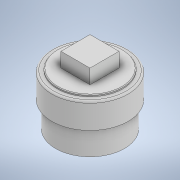
# Autodesk Inventor part: 4in Cleanout Adapter w Plug
Saved by Autodesk Inventor 2020 (Build 240168000, 168)
## iProperties
Created: 2020-01-08
Part Number: 4in Cleanout Adapter w Plug
Material: Generic
Document SubType Name: Modeling
Designer: ellio
Density: 1 g/cm^3
Appearance: Default
Author: ellio
Autodesk Inventor part; units mm, degrees
ref_plane "YZ Plane" through (0, 0, 0) normal (1, 0, 0) x (0, 1, 0)
ref_plane "XZ Plane" through (0, 0, 0) normal (0, 1, 0) x (-1, 0, 0)
ref_plane "XY Plane" through (0, 0, 0) normal (0, 0, 1) x (1, 0, 0)
sketch "Sketch1" plane through (0, 0, 0) normal (0, 1, 0) x (-1, 0, 0)
  circle A0 centre (0, 0) radius 53.975
  circle A1 centre (0, 0) radius 60.325
  dimension "d0" = 107.95
  dimension "d1" = 120.65
  constraints: 2 centre point, 2 coincident
  measures "d0" diameter of A0
  measures "d1" diameter of A1
extrude "Extrusion1" add sketch "Sketch1" along normal blind 44.45
sketch "Sketch2" plane through (0, 44.45, 0) normal (0, 1, 0) x (1, 0, 0)
  circle A0 centre (0, 0) radius 66.675
  dimension "d4" = 133.35
  constraints: 1 centre point, 1 coincident
  measures "d4" diameter of A0
extrude "Extrusion2" add sketch "Sketch2" along normal blind 44.45
sketch "Sketch3" plane through (0, 44.45, 0) normal (0, -1, 0) x (1, 0, 0)
  circle A0 centre (0, 0) radius 53.975
  dimension "d7" = 107.95
  constraints: 1 centre point, 1 coincident
  measures "d7" diameter of A0
extrude "Extrusion3" cut sketch "Sketch3" against normal blind 31.75
sketch "Sketch4" plane through (0, 88.9, 0) normal (0, 1, 0) x (1, 0, 0)
  circle A0 centre (0, 0) radius 57.15
  dimension "d10" = 114.3
  constraints: 1 centre point, 1 coincident
  measures "d10" diameter of A0
extrude "Extrusion4" add sketch "Sketch4" along normal blind 3.175
sketch "Sketch5" plane through (0, 92.075, 0) normal (0, 1, 0) x (1, 0, 0)
  line L0 (-25.4, -25.4) -> (25.4, -25.4)
  line L1 (25.4, -25.4) -> (25.4, 25.4)
  line L2 (25.4, 25.4) -> (-25.4, 25.4)
  line L3 (-25.4, 25.4) -> (-25.4, -25.4)
  point P0 (0, 0)
  dimension "d13" = 50.8
  dimension "d14" = 50.8
  constraints: 8 end point, 2 parallel, 1 horizontal, 1 perpendicular
  measures "d13" distance of L2.end L1.end
  measures "d14" distance of L1.end L0.end
extrude "Extrusion5" add sketch "Sketch5" along normal blind 25.4
fillet "Fillet1" radius 3.175 1 edges at (-66.675, 88.9, 0)
fillet "Fillet2" radius 1.27 1 edges at (-57.15, 92.075, 0)
body "Solid1"
